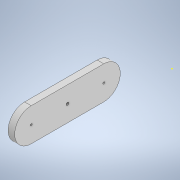
# Autodesk Inventor part: Second Arm half scale
Saved by Autodesk Inventor 2020.2 (Build 242310000, 310)
## iProperties
Created: 2020-03-31
Part Number: Second Arm half scale
Material: Generic
Document SubType Name: Modeling
Designer: Amaan Khalid
Density: 1 g/cm^3
Appearance: Default
Author: Amaan Khalid
Autodesk Inventor part; units mm, degrees
ref_plane "YZ Plane" through (0, 0, 0) normal (1, 0, 0) x (0, 1, 0)
ref_plane "XZ Plane" through (0, 0, 0) normal (0, 1, 0) x (-1, 0, 0)
ref_plane "XY Plane" through (0, 0, 0) normal (0, 0, 1) x (1, 0, 0)
sketch "Sketch1" plane through (0, 0, 0) normal (1, 0, 0) x (0, 1, 0)
  arc A0 (4.9966, 65.5864) -> (36.7466, 65.5864) centre (20.8716, 65.5864) ccw
  line L0 (36.7466, 65.5864) -> (36.7466, 100.5114)
  line L1 (4.9966, 65.5864) -> (4.9966, 100.5114)
  arc A1 (36.7466, 135.4364) -> (4.9966, 135.4364) centre (20.8716, 135.4364) ccw
  line L2 (36.7466, 135.4364) -> (36.7466, 100.5114)
  line L3 (4.9966, 135.4364) -> (4.9966, 100.5114)
  circle A2 centre (20.8716, 135.4364) radius 0.9144
  circle A3 centre (20.8716, 65.5864) radius 0.9144
  dimension "d3" = 1.8288
  dimension "d4" = 1.8288
  constraints: 8 end point, 4 centre point, 4 point on circle, 2 coincident, 2 vertical
  measures "d3" diameter of A2
  measures "d4" diameter of A3
extrude "Extrusion1" add sketch "Sketch1" along normal blind 6.35
sketch "Sketch2" plane through (6.35, 0, 0) normal (1, 0, 0) x (0, 0, -1)
  point P0 (0, 0)
sketch "Sketch5" plane through (6.35, 0, 0) normal (1, 0, 0) x (0, 0, -1)
  circle A0 centre (-135.4364, 20.8716) radius 0.9144 projected
  circle A1 centre (-65.5864, 20.8716) radius 0.9144 projected
  circle A2 centre (-100.5114, 20.8716) radius 1.27
  point P0 (0, 0)
  dimension "d18" = 2.54
  constraints: 1 centre point
  measures "d18" diameter of A2
extrude "Extrusion4" cut sketch "Sketch5" against normal blind 2.9972 contours A2
body "Solid1"
